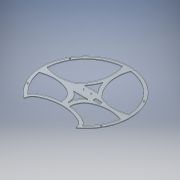
# Autodesk Inventor part: Handle
Saved by Autodesk Inventor 2017 (Build 210142000, 142)
## iProperties
Created: 2019-03-16
Part Number: Handle
Material: Generic
Document SubType Name: Modeling
Designer: Nicholas Cresswell
Density: 1 g/cm^3
Appearance: Clear
Author: Nicholas Cresswell
Autodesk Inventor part; units mm, degrees
ref_plane "YZ Plane" through (0, 0, 0) normal (1, 0, 0) x (0, 1, 0)
ref_plane "XZ Plane" through (0, 0, 0) normal (0, 1, 0) x (-1, 0, 0)
ref_plane "XY Plane" through (0, 0, 0) normal (0, 0, 1) x (1, 0, 0)
sketch "Sketch1" plane through (0, 0, 0) normal (0, 0, 1) x (1, 0, 0)
  arc A0 (62.337932, -109.534374) -> (-62.338968, -109.533936) centre (-0.000221, -25.04158) ccw
  arc A1 (-62.338968, -109.533936) -> (-60.750413, -108.830564) centre (-61.745267, -108.72925) ccw
  arc A2 (-50.002249, -92.706201) -> (-60.750413, -108.830564) centre (-40.131347, -110.93037) ccw
  arc A3 (50.001023, -92.708465) -> (-50.002249, -92.706201) centre (-0.002704, -185.038808) ccw
  arc A4 (60.74939, -108.831068) -> (62.337932, -109.534374) centre (61.744237, -108.729684) ccw
  arc A5 (60.74939, -108.831068) -> (50.001023, -92.708465) centre (40.131464, -110.932229) ccw
  arc A6 (53.872108, -86.277709) -> (-53.749901, -86.208202) centre (-0.002704, -185.038808) ccw construction
  arc A7 (65.047278, -97.671277) -> (53.872108, -86.277709) centre (40.131464, -110.932229) ccw construction
  arc A8 (65.047278, -97.671277) -> (-65.048011, -97.671016) centre (-0.000221, -25.04158) ccw construction
  arc A9 (-53.749901, -86.208202) -> (-65.048011, -97.671016) centre (-40.131347, -110.93037) ccw construction
  arc A10 (65.047278, -97.671277) -> (-65.048011, -97.671016) centre (-0.000221, -25.04158) ccw
  arc A11 (-53.749901, -86.208202) -> (-65.048011, -97.671016) centre (-40.131347, -110.93037) ccw
  arc A12 (53.872108, -86.277709) -> (-53.749901, -86.208202) centre (-0.002704, -185.038808) ccw
  arc A13 (65.047278, -97.671277) -> (53.872108, -86.277709) centre (40.131464, -110.932229) ccw
  point P0 (0, 0)
  constraints: 16 point on circle, 8 centre point, 6 concentric, 4 coincident
extrude "Extrusion1" add sketch "Sketch1" along normal blind 2
fillet "Fillet1" radius 1 2 edges at (-65.048, -97.671, 1) (65.0473, -97.6713, 1)
sketch "Sketch2" plane through (0, 0, 2) normal (0, 0, 1) x (1, 0, 0)
  arc A0 (65.981978, -96.82319) -> (-65.982771, -96.822866) centre (-0.000221, -25.04158) ccw construction
  circle A1 centre (-0.000221, -25.04158) radius 101.25 construction
  line L0 (-0.000221, -25.04158) -> (-87.685293, 25.58342) construction
  line L1 (-0.000221, -25.04158) -> (101.249779, -25.04158) construction
  line L2 (-0.000221, -25.04158) -> (87.684851, 25.58342) construction
  line L3 (-0.000221, -25.04158) -> (-87.685293, -75.66658) construction
  line L4 (-0.000221, -25.04158) -> (101.249779, -25.04158) construction
  line L5 (-0.000221, -25.04158) -> (87.684851, -75.66658) construction
  line L6 (-0.000221, -25.04158) -> (101.249779, -25.04158) construction
  line L7 (-0.000221, -25.04158) -> (101.249779, -25.04158) construction
  circle A2 centre (87.684851, 25.58342) radius 1.5
  circle A3 centre (87.684851, -75.66658) radius 1.5
  circle A4 centre (-87.685293, -75.66658) radius 1.5
  circle A5 centre (-87.685293, 25.58342) radius 1.5
  line L8 (-0.000221, -25.04158) -> (-0.000221, -72.538808) construction
  arc A6 (53.872108, -86.277709) -> (-53.749901, -86.208202) centre (-0.002704, -185.038808) ccw construction
  line L9 (-0.000221, -72.538808) -> (-0.000221, -80.037547) construction
  arc A7 (50.001023, -92.708465) -> (-50.002249, -92.706201) centre (-0.002704, -185.038808) ccw construction
  circle A8 centre (-0.000221, -76.288177) radius 1.5
  point P0 (0, 0)
  dimension "d7" = 202.5
  dimension "d8" = 150
  dimension "d9" = 150
  dimension "d10" = 30
  dimension "d14" = 3
  dimension "d15" = 3
  dimension "d16" = 3
  dimension "d17" = 3
  dimension "d18" = 3
  constraints: 20 end point, 6 centre point, 6 point on circle, 5 coincident, 4 horizontal, 3 equal length, 2 vertical, 1 midpoint
  measures "d7" diameter of A1
  measures "d8" angle of L1 L0
  measures "d9" angle of L3 L4
  measures "d10" angle of L5 L6
  measures "d14" diameter of A2
  measures "d15" diameter of A3
  measures "d16" diameter of A4
  measures "d17" diameter of A5
  measures "d18" diameter of A8
extrude "Extrusion3" cut sketch "Sketch2" against normal up to next contours A2 | A3 | A4 | A5
sketch "Sketch3" plane through (0, 0, 2) normal (0, 0, 1) x (1, 0, 0)
  arc A0 (10.069954, -72.990642) -> (-9.930046, -72.977674) centre (-0.002704, -185.038808) ccw
  line L0 (0.08586, -41.541785) -> (-29.91414, -41.541785) construction
  line L1 (-29.91414, -41.541785) -> (30.08586, -41.541785) construction
  line L2 (30.08586, -41.541785) -> (30.08586, -17.041498) construction
  line L3 (30.08586, -17.041498) -> (-29.91414, -17.041498) construction
  line L4 (-29.91414, -17.041498) -> (-29.91414, -41.541785) construction
  line L5 (30.08586, -29.291641) -> (97.407104, -29.291641) construction
  line L6 (30.08586, -29.291641) -> (97.407104, -29.291641) construction
  line L7 (-29.91414, -29.291641) -> (-97.407546, -29.291641) construction
  line L8 (0.069954, -72.538832) -> (0.213372, 161.863698) construction
  line L9 (-29.91414, -29.291641) -> (30.08586, -29.291641) construction
  line L10 (0.08586, -29.291641) -> (-8.80414, -29.291641) construction
  line L11 (0.08586, -29.291641) -> (8.97586, -29.291641) construction
  line L12 (-8.80414, -29.291641) -> (8.97586, -29.291641)
  arc A1 (30.08586, -41.541785) -> (10.069954, -72.990642) centre (45.069483, -73.172325) ccw
  arc A2 (-9.930046, -72.977674) -> (-29.91414, -41.541785) centre (-44.929585, -73.15723) ccw
  arc A3 (96.452803, -39.291641) -> (30.08586, -41.541785) centre (65.920739, -118.618769) ccw
  line L13 (-97.407546, -29.291641) -> (-87.407546, -29.291641) construction
  arc A4 (-29.91414, -41.541785) -> (-96.453245, -39.291641) centre (-65.827012, -118.58246) ccw
  line L14 (-97.407546, -29.291641) -> (-87.407546, -29.291641) construction
  arc A5 (-97.330526, -19.291641) -> (-29.91414, -17.041498) centre (-66.225021, 59.812389) ccw
  arc A6 (30.08586, -17.041498) -> (97.329893, -19.288417) centre (66.314736, 59.85108) ccw
  arc A7 (10.15867, 71.927729) -> (30.08586, -17.041498) centre (90.129276, 43.123178) ccw
  arc A8 (-29.91414, -17.041498) -> (-9.84133, 71.960495) centre (-89.841664, 43.238613) ccw
  line L15 (0.10391, -17.041498) -> (0.106969, -12.041499)
  line L16 (0.106969, -12.041499) -> (0.123795, 15.458496) construction
  line L17 (0.106969, -12.041499) -> (15.606969, -12.041499) construction
  line L18 (0.106969, -12.041499) -> (-15.393031, -12.041499) construction
  arc A9 (-15.393031, -12.041499) -> (0.123795, 15.458496) centre (-80.375006, 42.75214) ccw construction
  arc A10 (0.123795, 15.458496) -> (15.606969, -12.041499) centre (80.645215, 42.685337) ccw construction
  line L19 (-15.393031, -12.041499) -> (15.606969, -12.041499)
  arc A11 (-15.393031, -12.041499) -> (0.123795, 15.458496) centre (-80.375006, 42.75214) ccw
  arc A12 (0.123795, 15.458496) -> (15.606969, -12.041499) centre (80.645215, 42.685337) ccw
  line L20 (0.08586, -41.541785) -> (0.08586, -46.541785)
  line L21 (0.08586, -41.541785) -> (5.08586, -41.541785) construction
  arc A13 (96.452803, -39.291641) -> (97.329893, -19.288417) centre (-0.000221, -25.04158) ccw
  arc A14 (10.15867, 71.927729) -> (-9.84133, 71.960495) centre (-0.000221, -25.04158) ccw
  arc A15 (-97.330526, -19.291641) -> (-96.453245, -39.291641) centre (-0.000221, -25.04158) ccw
  line L22 (-29.91414, -29.291641) -> (-29.91414, -34.291641) construction
  line L23 (8.97586, -29.291641) -> (8.97586, -21.291641)
  line L24 (-8.80414, -29.291641) -> (-8.80414, -21.291641)
  circle A16 centre (-8.80414, -21.291641) radius 1
  circle A17 centre (8.97586, -21.291641) radius 1
  point P0 (0, 0)
  dimension "d30" = 30
  dimension "d31" = 60
  dimension "d43" = 8.89
  dimension "d44" = 180
  dimension "d46" = 17.78
  dimension "d55" = 35
  dimension "d56" = 35
  dimension "d60" = 85
  dimension "d63" = 85
  dimension "d66" = 85
  dimension "d67" = 85
  dimension "d72" = 85
  dimension "d73" = 85
  dimension "d74" = 5
  dimension "d75" = 27.5
  dimension "d76" = 15.5
  dimension "d77" = 15.5
  dimension "d78" = 85
  dimension "d79" = 85
  dimension "d80" = 5
  dimension "d81" = 90
  dimension "d89" = 5
  dimension "d109" = 8
  dimension "d110" = 8
  dimension "d111" = 2
  dimension "d112" = 2
  constraints: 50 end point, 34 point on circle, 18 centre point, 10 horizontal, 5 point on line, 4 coincident, 3 midpoint, 3 perpendicular, 3 vertical, 2 collinear, 2 concentric, 2 equal length
  measures "d30" distance of L0.start L0.end
  measures "d31" distance of L0.end L1.end
  measures "d43" distance of L10.start L10.end
  measures "d44" angle of L10 L11
  measures "d46" distance of L12.start L11.end
  measures "d55" radius of A1
  measures "d56" radius of A2
  measures "d60" radius of A3
  measures "d63" radius of A4
  measures "d66" radius of A5
  measures "d67" radius of A6
  measures "d72" radius of A7
  measures "d73" radius of A8
  measures "d74" distance of L15.start L15.end
  measures "d75" distance of L15.end L16.end
  measures "d76" distance of L15.end L17.end
  measures "d77" distance of L15.end L18.end
  measures "d78" radius of A9
  measures "d79" radius of A10
  measures "d80" distance of L0.start L20.end
  measures "d81" angle of L20 L21
  measures "d89" distance of L7.start L22.end
  measures "d109" distance of L23.start L23.end
  measures "d110" distance of L12.start L24.end
  measures "d111" diameter of A16
  measures "d112" diameter of A17
sketch "Sketch6" plane through (0, 0, 2) normal (0, 0, 1) x (1, 0, 0)
  arc A0 (53.872108, -86.277709) -> (-53.749901, -86.208202) centre (-0.002704, -185.038808) ccw
  arc A1 (-53.749901, -86.208202) -> (-64.444618, -96.59456) centre (-40.131347, -110.93037) ccw
  arc A2 (-65.982771, -96.822866) -> (-64.444618, -96.59456) centre (-65.306027, -96.086648) ccw
  arc A3 (65.981978, -96.82319) -> (-65.982771, -96.822866) centre (-0.000221, -25.04158) ccw
  arc A4 (64.443859, -96.594932) -> (65.981978, -96.82319) centre (65.305237, -96.086968) ccw
  arc A5 (64.443859, -96.594932) -> (53.872108, -86.277709) centre (40.131464, -110.932229) ccw
  circle A6 centre (-87.685293, -75.66658) radius 1.5
  circle A7 centre (87.684851, 25.58342) radius 1.5
  circle A8 centre (87.684851, -75.66658) radius 1.5
  circle A9 centre (-87.685293, 25.58342) radius 1.5
  arc A10 (62.337932, -109.534374) -> (-62.338968, -109.533936) centre (-0.000221, -25.04158) ccw
  arc A11 (-62.338968, -109.533936) -> (-60.750413, -108.830564) centre (-61.745267, -108.72925) ccw
  arc A12 (-50.002249, -92.706201) -> (-60.750413, -108.830564) centre (-40.131347, -110.93037) ccw
  arc A13 (50.001023, -92.708465) -> (-50.002249, -92.706201) centre (-0.002704, -185.038808) ccw
  arc A14 (60.74939, -108.831068) -> (50.001023, -92.708465) centre (40.131464, -110.932229) ccw
  arc A15 (60.74939, -108.831068) -> (62.337932, -109.534374) centre (61.744237, -108.729684) ccw
  line L0 (-8.80414, -29.291641) -> (8.97586, -29.291641)
  line L1 (0.08586, -29.291641) -> (20.08586, -29.291641)
  line L2 (20.08586, -29.291641) -> (25.08586, -29.291641)
  line L3 (25.08586, -29.291641) -> (25.08586, -26.291641)
  line L4 (25.08586, -26.291641) -> (25.08586, -32.291641)
  line L5 (25.08586, -32.291641) -> (40.08586, -32.291641)
  line L6 (40.08586, -32.291641) -> (40.08586, -26.291641)
  line L7 (40.08586, -26.291641) -> (25.08586, -26.291641)
  point P0 (0, 0)
  dimension "d101" = 20
  dimension "d102" = 5
  dimension "d103" = 3
  dimension "d104" = 6
  dimension "d105" = 15
  dimension "d106" = 6
  constraints: 16 end point, 3 horizontal, 2 perpendicular, 1 midpoint, 1 point on line, 1 vertical
  measures "d101" distance of L1.start L1.end
  measures "d102" distance of L1.end L2.end
  measures "d103" distance of L2.end L3.end
  measures "d104" distance of L3.end L4.end
  measures "d105" distance of L4.end L5.end
  measures "d106" distance of L5.end L6.end
extrude "Extrusion9" add sketch "Sketch3" against normal blind 2
extrude "Extrusion10" cut sketch "Sketch6" against normal blind 2 contours L3 L7 L6 L5 L4
sketch "Sketch7" plane through (0, 0, 2) normal (0, 0, 1) x (1, 0, 0)
  line L0 (40.08586, -32.291641) -> (25.08586, -32.291641)
  line L1 (25.08586, -32.291641) -> (25.08586, -26.291641)
  line L2 (25.08586, -26.291641) -> (40.08586, -26.291641)
  line L3 (40.08586, -26.291641) -> (40.08586, -32.291641)
  arc A0 (-9.930046, -72.977674) -> (-53.749901, -86.208202) centre (-0.002704, -185.038808) ccw
  arc A1 (-53.749901, -86.208202) -> (-64.444618, -96.59456) centre (-40.131347, -110.93037) ccw
  arc A2 (-65.982771, -96.822866) -> (-64.444618, -96.59456) centre (-65.306027, -96.086648) ccw
  arc A3 (-96.453245, -39.291641) -> (-65.982771, -96.822866) centre (-0.000221, -25.04158) ccw
  arc A4 (-29.91414, -41.541785) -> (-96.453245, -39.291641) centre (-65.827012, -118.58246) ccw
  arc A5 (-9.930046, -72.977674) -> (-29.91414, -41.541785) centre (-44.929585, -73.15723) ccw
  arc A6 (30.08586, -41.541785) -> (10.069954, -72.990642) centre (45.069483, -73.172325) ccw
  arc A7 (96.452803, -39.291641) -> (30.08586, -41.541785) centre (65.920739, -118.618769) ccw
  arc A8 (65.981978, -96.82319) -> (96.452803, -39.291641) centre (-0.000221, -25.04158) ccw
  arc A9 (64.443859, -96.594932) -> (65.981978, -96.82319) centre (65.305237, -96.086968) ccw
  arc A10 (64.443859, -96.594932) -> (53.872108, -86.277709) centre (40.131464, -110.932229) ccw
  arc A11 (53.872108, -86.277709) -> (10.069954, -72.990642) centre (-0.002704, -185.038808) ccw
  arc A12 (30.08586, -17.041498) -> (97.329893, -19.288417) centre (66.314736, 59.85108) ccw
  arc A13 (10.15867, 71.927729) -> (30.08586, -17.041498) centre (90.129276, 43.123178) ccw
  arc A14 (97.329893, -19.288417) -> (10.15867, 71.927729) centre (-0.000221, -25.04158) ccw
  circle A15 centre (-8.80414, -21.291641) radius 1
  circle A16 centre (8.97586, -21.291641) radius 1
  line L4 (15.606969, -12.041499) -> (-15.393031, -12.041499)
  arc A17 (-15.393031, -12.041499) -> (0.123795, 15.458496) centre (-80.375006, 42.75214) ccw
  arc A18 (0.123795, 15.458496) -> (15.606969, -12.041499) centre (80.645215, 42.685337) ccw
  circle A19 centre (-87.685293, -75.66658) radius 1.5
  circle A20 centre (87.684851, 25.58342) radius 1.5
  circle A21 centre (87.684851, -75.66658) radius 1.5
  circle A22 centre (-87.685293, 25.58342) radius 1.5
  arc A23 (-29.91414, -17.041498) -> (-9.84133, 71.960495) centre (-89.841664, 43.238613) ccw
  arc A24 (-97.330526, -19.291641) -> (-29.91414, -17.041498) centre (-66.225021, 59.812389) ccw
  arc A25 (-9.84133, 71.960495) -> (-97.330526, -19.291641) centre (-0.000221, -25.04158) ccw
  arc A26 (62.337932, -109.534374) -> (-62.338968, -109.533936) centre (-0.000221, -25.04158) ccw
  arc A27 (-62.338968, -109.533936) -> (-60.750413, -108.830564) centre (-61.745267, -108.72925) ccw
  arc A28 (-50.002249, -92.706201) -> (-60.750413, -108.830564) centre (-40.131347, -110.93037) ccw
  arc A29 (50.001023, -92.708465) -> (-50.002249, -92.706201) centre (-0.002704, -185.038808) ccw
  arc A30 (60.74939, -108.831068) -> (50.001023, -92.708465) centre (40.131464, -110.932229) ccw
  arc A31 (60.74939, -108.831068) -> (62.337932, -109.534374) centre (61.744237, -108.729684) ccw
  line L5 (15.606969, -12.041499) -> (-15.393031, -12.041499)
  line L6 (0.106969, -12.041499) -> (0.106969, -37.041499)
  line L7 (-16.848413, -37.041499) -> (17.062352, -37.041499)
  line L8 (0.106969, -37.041499) -> (0.106969, -67.041499)
  arc A32 (0.106969, -67.041499) -> (-16.848413, -37.041499) centre (-34.893029, -67.031361) ccw
  arc A33 (17.062352, -37.041499) -> (0.106969, -67.041499) centre (35.106968, -67.031361) ccw
  point P0 (0, 0)
  dimension "d117" = 25
  dimension "d118" = 30
  dimension "d119" = 35
  dimension "d120" = 35
  dimension "d123" = 25
  constraints: 6 end point, 4 point on circle, 2 centre point, 2 vertical, 1 horizontal, 1 midpoint
  measures "d117" distance of L6.start L6.end
  measures "d118" distance of L6.end L8.end
  measures "d119" radius of A32
  measures "d120" radius of A33
  measures "d123" distance between parallel lines of L4 L7
sketch "Sketch7 outline for Extrusion11" plane through (0, 0, 2) normal (0, 0, 1) x (1, 0, 0)
  arc A0 (-16.848413, -37.041499) -> (0.106969, -67.041499) centre (-34.893029, -67.031361) cw
  line L0 (17.062352, -37.041499) -> (-16.848413, -37.041499)
  arc A1 (0.106969, -67.041499) -> (17.062352, -37.041499) centre (35.106968, -67.031361) cw
extrude "Extrusion11" cut sketch "Sketch7 outline for Extrusion11" against normal blind 2
body "Solid1"
